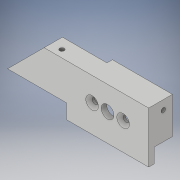
# Autodesk Inventor part: mocowanie_silnika_wariant1
Saved by Autodesk Inventor 2019 (Build 230136000, 136)
## iProperties
Created: 2019-11-17
Part Number: mocowanie_silnika_wariant1
Material: Generic
Document SubType Name: Modeling
Designer: Michal
Density: 1 g/cm^3
Appearance: Default
Author: Michal
Autodesk Inventor part; units mm, degrees
ref_plane "YZ Plane" through (0, 0, 0) normal (1, 0, 0) x (0, 1, 0)
ref_plane "XZ Plane" through (0, 0, 0) normal (0, 1, 0) x (-1, 0, 0)
ref_plane "XY Plane" through (0, 0, 0) normal (0, 0, 1) x (1, 0, 0)
sketch "Sketch1" plane through (0, 0, 0) normal (0, 1, 0) x (-1, 0, 0)
  line L0 (0, 0) -> (81.5, 0)
  line L1 (81.5, 0) -> (81.5, -13)
  line L2 (81.5, -13) -> (0, -13)
  line L3 (0, -13) -> (0, 0)
  dimension "d0" = 81.5
  dimension "d1" = 13
  constraints: 8 end point, 2 parallel, 1 horizontal, 1 perpendicular
  measures "d0" distance of L1.end L2.end
  measures "d1" distance of L0.end L1.end
extrude "Extrusion1" add sketch "Sketch1" along normal blind 30
sketch "Sketch2" plane through (0, 0, -13) normal (0, 0, -1) x (-1, 0, 0)
  line L0 (0, 0) -> (0, 30) projected
  line L1 (0, 0) -> (81.5086, 0)
  line L2 (81.5086, 0) -> (81.5086, 8)
  line L3 (81.5086, 8) -> (0, 8)
  line L4 (0, 8) -> (0, 0)
  line L5 (81.5, 0) -> (81.5, 30) projected
  line L6 (81.5, 0) -> (22.5, 0)
  line L7 (0, 0) -> (81.5, 0) projected
  line L8 (22.5, 0) -> (22.5, 15)
  circle A0 centre (22.5, 15) radius 12.5
  dimension "d4" = 81.5086
  dimension "d5" = 8
  dimension "d6" = 59
  dimension "d7" = 15
  dimension "d8" = 25
  constraints: 12 end point, 2 parallel, 2 perpendicular, 1 centre point, 1 coincident, 1 horizontal, 1 point on line
  measures "d4" distance of L3.end L2.end
  measures "d5" distance of L2.end L1.end
  measures "d6" distance of L5.start L6.end
  measures "d7" distance of L6.end L8.end
  measures "d8" diameter of A0
extrude "Extrusion2" cut sketch "Sketch2" against normal blind 10
sketch "Sketch3" plane through (-81.5, 0, 0) normal (0, 0, 1) x (1, 0, 0)
  line L0 (0, 8) -> (0, 30) projected
  line L1 (0, 30) -> (0, 8)
  line L2 (0, 30) -> (22, 30)
  line L3 (0, 30) -> (81.5, 30) projected
  line L4 (22, 30) -> (0, 8)
  line L5 (81.5, 0) -> (81.5, 8) projected
  line L6 (81.5, 0) -> (36.5, 0)
  line L7 (0, 0) -> (81.5, 0) projected
  line L8 (48.6438, 8) -> (0, 8) projected
  line L9 (36.5, 0) -> (0, 0)
  line L10 (0, 0) -> (0, 8)
  line L11 (0, 8) -> (36.5, 8)
  line L12 (36.5, 8) -> (36.5, 0)
  dimension "d11" = 22
  dimension "d12" = 45
  constraints: 16 end point, 4 point on line, 3 equal length, 1 horizontal, 1 perpendicular
  measures "d11" distance of L0.end L2.end
  measures "d12" distance of L5.start L6.end
extrude "Extrusion3" cut sketch "Sketch3" against normal blind 13
sketch "Sketch4" plane through (0, 30, 0) normal (0, 1, 0) x (1, 0, 0)
  line L0 (0, 0) -> (0, 13) projected
  line L1 (-59.5, 0) -> (-81.5, 0) projected
  line L2 (0, 13) -> (-81.5, 13)
  line L3 (-81.5, 13) -> (-81.5, 0)
  line L4 (-81.5, 0) -> (0, 0)
  line L5 (0, 0) -> (0, 13)
  constraints: 8 end point, 2 parallel, 1 horizontal, 1 perpendicular
extrude "Extrusion4" cut sketch "Sketch4" against normal blind 2
sketch "Sketch6" plane through (0, 0, -3) normal (0, 0, -1) x (-1, 0, 0)
  arc A0 (32.8562, 8) -> (12.1438, 8) centre (22.5, 15) ccw projected
  circle A1 centre (22.5, 15) radius 3.5
  point P0 (0, 0)
  dimension "d17" = 7
  constraints: 1 centre point, 1 coincident
  measures "d17" diameter of A1
extrude "Extrusion5" cut sketch "Sketch6" against normal blind 3
sketch "Sketch7" plane through (-45, 0, 0) normal (0, 0, 1) x (1, 0, 0)
  circle A0 centre (22.5, 15) radius 3.5 projected
  line L0 (22.5, 15) -> (31, 15)
  line L1 (22.5, 15) -> (14, 15)
  point P0 (45, 0)
  dimension "d20" = 8.5
  dimension "d21" = 8.5
  constraints: 4 end point, 2 horizontal
  measures "d20" distance of L0.start L0.end
  measures "d21" distance of L0.start L1.end
hole "Hole1" at (-14, 15, 0) at (-31, 15, 0) direction (0, 0, -1) diameter 3.4 end through all countersink diameter 6.9 countersink angle 89.954 clearance for "Countersunk Flat Head Screw ISO 2009/7046" size "M3" standard "ISO"
sketch "Sketch8" plane through (-32.8562, 8, -13) normal (0, -1, 0) x (1, 0, 0)
  line L0 (0, 0) -> (-48.6438, 0) projected
  line L1 (-48.6438, 0) -> (-36.6438, 0)
  line L2 (-36.6438, 0) -> (-36.6438, 8)
  line L3 (32.8562, 10) -> (32.8562, 0) projected
  line L4 (32.8562, 0) -> (32.8562, 5)
  line L5 (32.8562, 5) -> (27.8562, 5)
  point P0 (32.8562, 13)
  dimension "d82" = 8
  dimension "d83" = 5
  dimension "d84" = 5
  constraints: 8 end point, 2 perpendicular, 1 midpoint, 1 point on line
  measures "d82" distance of L1.end L2.end
  measures "d83" distance of L3.end L4.end
  measures "d84" distance of L4.end L5.end
hole "Hole2" at (-5, 8, -8) at (-69.5, 8, -5) direction (0, 1, 0) diameter 4.134 depth 5.6 tip angle 118 thread size "M5x0.8" class "6H" standard "ISO Metric profile"
sketch "Sketch9" plane through (0, 0, 0) normal (1, 0, 0) x (0, 0, -1)
  line L0 (8, 28) -> (8, 23)
  line L1 (0, 28) -> (13, 28) projected
  line L2 (8, 28) -> (13, 28)
  point P0 (0, 0)
  point P1 (13, 8)
  dimension "d40" = 5
  constraints: 4 end point, 1 collinear
  measures "d40" distance of L0.start L0.end
hole "Hole3" at (0, 23, -8) direction (-1, 0, 0) diameter 2.459 depth 9 tip angle 118 thread size "M3x0.5" class "6H" standard "ISO Metric profile"
sketch "Sketch10" plane through (0, 28, 0) normal (0, 1, 0) x (1, 0, 0)
  line L0 (-61.5, 0) -> (-61.5, 13) projected
  line L1 (-61.5, 0) -> (-61.5, 4)
  line L2 (-61.5, 4) -> (-51.5, 4)
  point P0 (0, 0)
  dimension "d76" = 4
  dimension "d77" = 10
  constraints: 4 end point, 1 perpendicular, 1 point on line
  measures "d76" distance of L0.start L1.end
  measures "d77" distance of L1.end L2.end
hole "Hole4" at (-51.5, 28, -4) direction (0, -1, 0) diameter 2.459 depth 9 tip angle 118 thread size "M3x0.5" class "6H" standard "ISO Metric profile"
sketch "Sketch12" plane through (-45, 0, 0) normal (0, 0, 1) x (1, 0, 0)
  line L0 (12.1438, 8) -> (-36.5, 8) projected
  line L1 (-36.5, 8) -> (-33.5, 8)
  line L2 (-16.5, 28) -> (45, 28) projected
  line L3 (-16.5, 28) -> (-13.5, 28)
  line L4 (-13.5, 28) -> (-33.5, 8)
  line L5 (-36.5, 8) -> (-16.5, 28)
  line L6 (-13.5, 28) -> (-12.257, 28)
  line L7 (45, 28) -> (-16.5, 28) projected
  line L8 (-12.257, 28) -> (-32.257, 8)
  line L9 (-33.5, 8) -> (-32.257, 8)
  point P0 (45, 0)
  dimension "d71" = 3
  dimension "d72" = 3
  dimension "d75" = 1.243
  constraints: 14 end point, 4 point on line, 1 collinear
  measures "d71" distance of L0.end L1.end
  measures "d72" distance of L2.start L3.end
  measures "d75" distance of L3.end L6.end
extrude "Extrusion6" cut sketch "Sketch12" against normal blind 25.4
sketch "Sketch13" plane through (-22.5, 15, -13) normal (0, 0, -1) x (-1, 0, 0)
  line L0 (10.3562, -7) -> (54.757, -7) projected
  line L1 (10.3562, -7) -> (47.3562, -7)
  line L2 (47.3562, -7) -> (47.3562, 0.4008)
  line L3 (34.757, 13) -> (54.757, -7) projected
  line L4 (34.757, 13) -> (-22.5, 13) projected
  line L5 (47.3562, 0.4008) -> (34.757, 13)
  line L6 (34.757, 13) -> (10.3562, 13)
  arc A0 (10.3562, -7) -> (-10.3562, -7) centre (0, 0) ccw projected
  line L7 (10.3562, -7) -> (10.3562, 13)
  line L8 (49.067, -7) -> (44.933, -7) projected
  line L9 (47.3562, -7) -> (49.067, -7)
  line L10 (49.067, -7) -> (49.067, -1.31)
  line L11 (47.3562, 0.4008) -> (49.067, -1.31)
  line L12 (54.757, -7) -> (34.757, 13) projected
  point P0 (-22.5, -15)
  dimension "d79" = 37
  constraints: 16 end point, 4 point on line, 2 collinear, 2 perpendicular, 1 vertical
  measures "d79" distance of L0.start L1.end
extrude "Extrusion7" cut sketch "Sketch13" against normal blind 3 contours A0 L7 L4 L3 L2 L0 | L7 A0 | L2 L3 L10 L0
sketch "Sketch11" plane through (-79.3785, 5.8785, -13) normal (-0.7071068, 0.7071068, 0) x (-0.7071068, -0.7071068, 0)
  line L0 (-31.2845, 3) -> (-31.2845, 13) projected
  line L1 (-3.0003, 0) -> (-11.0471, 0) projected
  point P0 (-51.9723, 13)
  point P1 (-25.9845, 7)
  dimension "d111" = 5.3
  dimension "d112" = 7
  measures "d111" distance from line of L0 point (-25.985, 7)
  measures "d112" distance from line of L1 point (-25.985, 7)
hole "Hole5" at (-61.0047, 24.2523, -6) direction (0.7071068, -0.7071068, 0) diameter 2.459 depth 10 tip angle 118 thread size "M3x0.5" class "6H" standard "ISO Metric profile"
body "Solid1"
